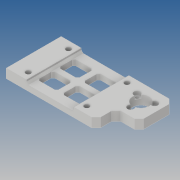
# Autodesk Inventor part: attache_moteur
Saved by Autodesk Inventor 2019 (Build 230136000, 136)
## iProperties
Created: 2020-07-07
Part Number: attache_moteur
Material: Générique
Document SubType Name: Modeling
Designer: Theo
Density: 1 g/cm^3
Appearance: Par défaut
Author: Theo
Autodesk Inventor part; units mm, degrees
ref_plane "YZ Plane" through (0, 0, 0) normal (1, 0, 0) x (0, 1, 0)
ref_plane "XZ Plane" through (0, 0, 0) normal (0, 1, 0) x (-1, 0, 0)
ref_plane "XY Plane" through (0, 0, 0) normal (0, 0, 1) x (1, 0, 0)
sketch "Esquisse1" plane through (0, 0, 0) normal (0, 1, 0) x (-1, 0, 0)
  line L0 (0, 0) -> (123, 0)
  line L1 (123, 0) -> (123, 60)
  line L2 (123, 60) -> (0, 60)
  line L3 (0, 60) -> (0, 0)
  dimension "d1" = 123
  dimension "d2" = 60
  constraints: 8 end point, 2 parallel, 1 horizontal, 1 perpendicular
  measures "d1" distance of L0.start L0.end
  measures "d2" distance of L2.end L0.start
extrude "Extrusion1" add sketch "Esquisse1" along normal blind 10
sketch "Esquisse2" plane through (0, 10, 0) normal (0, 1, 0) x (1, 0, 0)
  circle A0 centre (-18, -18) radius 9
  line L0 (0, 0) -> (-123, 0) projected
  line L1 (-123, 0) -> (-123, -60) projected
  line L2 (-123, -60) -> (0, -60) projected
  line L3 (0, -60) -> (0, 0) projected
  line L4 (-29, -9) -> (-7, -9) construction
  line L5 (-7, -9) -> (-7, -56) construction
  line L6 (-7, -56) -> (-29, -56) construction
  line L7 (-29, -56) -> (-29, -9) construction
  dimension "d5" = 18
  dimension "d7" = 18
  dimension "d9" = 18
  dimension "d27" = 22
  dimension "d28" = 11
  dimension "d29" = 9
  dimension "d30" = 47
  dimension "d31" = 7
  dimension "d44" = 9
  constraints: 8 end point, 2 parallel, 1 centre point, 1 horizontal, 1 perpendicular
  measures "d5" diameter of A0
  measures "d7" distance from line of L3 A0.centre
  measures "d9" distance from line of A0.centre L0
  measures "d27" distance of L4.start L4.end
  measures "d28" horizontal distance of L4.end A0.centre
  measures "d29" distance from line of L4 A0.centre
  measures "d30" distance of L6.end L4.start
  measures "d31" distance between parallel lines of L3 L5
  measures "d44" distance between parallel lines of L0 L4
extrude "Extrusion2" cut sketch "Esquisse2" against normal up to surface (10 mm away) contours A0
sketch "Esquisse4" plane through (0, 10, 0) normal (0, 1, 0) x (1, 0, 0)
  circle A0 centre (-18, -18) radius 9 projected
  line L0 (0, 0) -> (-123, 0) projected
  line L1 (-123, 0) -> (-123, -60) projected
  line L2 (-123, -60) -> (0, -60) projected
  line L3 (0, -60) -> (0, 0) projected
  point P0 (-18, -29)
  dimension "d16" = 11
  constraints: 1 vertical alignment
  measures "d16" distance of point (-18, -29) A0.centre
hole "Perçage1" at (-18, 10, 29) direction (0, -1, 0) diameter 3.4 end through all counterbore diameter 7 counterbore depth 4 clearance for "Vis d'assemblage à tête hexagonale ISO 24017" size "M3" standard "ISO"
pattern_circular "Réseau circulaire1" count 3 over 360 about axis through (-18, 10, 18) along (0, -1, 0) of "Perçage1"
sketch "Esquisse5" plane through (0, 10, 0) normal (0, 1, 0) x (1, 0, 0)
  arc A0 (-9.2451, -15.9139) -> (-11.816, -11.4611) centre (-8.4737, -12.5) ccw projected
  arc A1 (-15.4291, -26.625) -> (-9.2451, -15.9139) centre (-18, -18) ccw projected
  arc A2 (-20.5709, -26.625) -> (-15.4291, -26.625) centre (-18, -29) ccw projected
  arc A3 (-26.7549, -15.9139) -> (-20.5709, -26.625) centre (-18, -18) ccw projected
  arc A4 (-24.184, -11.4611) -> (-26.7549, -15.9139) centre (-27.5263, -12.5) ccw projected
  arc A5 (-11.816, -11.4611) -> (-24.184, -11.4611) centre (-18, -18) ccw projected
  line L0 (0, 0) -> (-123, 0) projected
  line L1 (-123, 0) -> (-123, -60) projected
  line L2 (-123, -60) -> (0, -60) projected
  line L3 (0, -60) -> (0, 0) projected
  line L4 (-29, -18.7209) -> (-29, -39.8718) construction
  point P0 (-43, -8)
  point P1 (-43, -52)
  point P2 (-107, -8)
  point P3 (-107, -52)
  dimension "d32" = 11
  dimension "d33" = 14
  dimension "d34" = 8
  dimension "d35" = 8
  dimension "d36" = 16
  constraints: 2 end point, 2 horizontal alignment, 2 vertical alignment, 1 vertical
  measures "d32" distance from line of L4 A1.centre
  measures "d33" distance from line of point (-43, -8) L4
  measures "d34" distance from line of L0 point (-43, -8)
  measures "d35" distance from line of L2 point (-43, -52)
  measures "d36" distance from line of L1 point (-107, -8)
hole "Perçage2" at (-43, 10, 8) at (-43, 10, 52) at (-107, 10, 8) at (-107, 10, 52) direction (0, -1, 0) diameter 5.5 end through all clearance for "Vis d'assemblage à tête hexagonale ISO 24017" size "M5" standard "ISO"
sketch "Esquisse6" plane through (0, 10, 0) normal (0, 1, 0) x (1, 0, 0)
  circle A0 centre (-107, -8) radius 2.75 projected
  circle A1 centre (-43, -8) radius 2.75 projected
  circle A2 centre (-43, -52) radius 2.75 projected
  circle A3 centre (-107, -52) radius 2.75 projected
  arc A4 (-9.2451, -15.9139) -> (-11.816, -11.4611) centre (-8.4737, -12.5) ccw projected
  arc A5 (-15.4291, -26.625) -> (-9.2451, -15.9139) centre (-18, -18) ccw projected
  arc A6 (-20.5709, -26.625) -> (-15.4291, -26.625) centre (-18, -29) ccw projected
  arc A7 (-26.7549, -15.9139) -> (-20.5709, -26.625) centre (-18, -18) ccw projected
  arc A8 (-24.184, -11.4611) -> (-26.7549, -15.9139) centre (-27.5263, -12.5) ccw projected
  arc A9 (-11.816, -11.4611) -> (-24.184, -11.4611) centre (-18, -18) ccw projected
  line L0 (0, 0) -> (-123, 0) projected
  line L1 (-123, 0) -> (-123, -60) projected
  line L2 (-123, -60) -> (0, -60) projected
  line L3 (0, -60) -> (0, 0) projected
  line L4 (-99, -10) -> (-78, -10)
  line L5 (-78, -10) -> (-78, -27)
  line L6 (-78, -27) -> (-99, -27)
  line L7 (-99, -27) -> (-99, -10)
  line L8 (-72, -10) -> (-51, -10)
  line L9 (-51, -10) -> (-51, -27)
  line L10 (-51, -27) -> (-72, -27)
  line L11 (-72, -27) -> (-72, -10)
  line L12 (-72, -33) -> (-51, -33)
  line L13 (-51, -33) -> (-51, -50)
  line L14 (-51, -50) -> (-72, -50)
  line L15 (-72, -50) -> (-72, -33)
  line L16 (-99, -33) -> (-78, -33)
  line L17 (-78, -33) -> (-78, -50)
  line L18 (-78, -50) -> (-99, -50)
  line L19 (-99, -50) -> (-99, -33)
  dimension "d47" = 10
  dimension "d48" = 10
  dimension "d49" = 8
  dimension "d50" = 6
  dimension "d51" = 6
  dimension "d52" = 8
  constraints: 32 end point, 8 parallel, 6 point on line, 4 horizontal, 4 perpendicular, 2 collinear, 2 horizontal alignment, 2 vertical alignment
  measures "d47" distance between parallel lines of L0 L4
  measures "d48" distance between parallel lines of L2 L18
  measures "d49" distance from line of L7 A0.centre
  measures "d50" distance between parallel lines of L6 L16
  measures "d51" distance between parallel lines of L11 L5
  measures "d52" distance from line of L9 A1.centre
extrude "Extrusion4" cut sketch "Esquisse6" against normal up to surface (10 mm away) contours L4 L5 L6 L7 | L8 L9 L10 L11 | L12 L13 L14 L15 | L16 L17 L18 L19
chamfer "Chanfrein1" distance 2 angle 45 16 edges at (-78, 5, 27) (-78, 5, 50) (-51, 5, 50) (-51, 5, 27) (-72, 5, 33) (-72, 5, 10) (-99, 5, 10) (-99, 5, 33) (-78, 5, 33) (-78, 5, 10) (-51, 5, 10) (-51, 5, 33) (-99, 5, 50) (-72, 5, 50) (-99, 5, 27) (-72, 5, 27)
chamfer "Chanfrein3" distance 5 angle 45 1 edges at (0, 5, 0)
sketch "Esquisse7" plane through (0, 10, 0) normal (0, 1, 0) x (1, 0, 0)
  line L0 (-5, 0) -> (-123, 0) projected
  line L1 (-101, 0) -> (-49, 0)
  line L2 (-49, 0) -> (-49, -60)
  line L3 (-49, -60) -> (-101, -60)
  line L4 (-101, -60) -> (-101, 0)
  line L5 (-51, -35) -> (-51, -48) projected
  line L6 (-53, -50) -> (-51, -48) projected
  line L7 (-53, -50) -> (-70, -50) projected
  line L8 (-72, -48) -> (-70, -50) projected
  line L9 (-72, -48) -> (-72, -35) projected
  line L10 (-70, -33) -> (-72, -35) projected
  line L11 (-70, -33) -> (-53, -33) projected
  line L12 (-51, -35) -> (-53, -33) projected
  line L13 (-80, -50) -> (-97, -50) projected
  line L14 (-99, -48) -> (-97, -50) projected
  line L15 (-99, -48) -> (-99, -35) projected
  line L16 (-97, -33) -> (-99, -35) projected
  line L17 (-97, -33) -> (-80, -33) projected
  line L18 (-78, -35) -> (-80, -33) projected
  line L19 (-78, -35) -> (-78, -48) projected
  line L20 (-80, -50) -> (-78, -48) projected
  line L21 (-51, -12) -> (-51, -25) projected
  line L22 (-53, -27) -> (-51, -25) projected
  line L23 (-53, -27) -> (-70, -27) projected
  line L24 (-72, -25) -> (-70, -27) projected
  line L25 (-72, -25) -> (-72, -12) projected
  line L26 (-70, -10) -> (-72, -12) projected
  line L27 (-70, -10) -> (-53, -10) projected
  line L28 (-51, -12) -> (-53, -10) projected
  line L29 (-80, -27) -> (-97, -27) projected
  line L30 (-99, -25) -> (-97, -27) projected
  line L31 (-99, -25) -> (-99, -12) projected
  line L32 (-97, -10) -> (-99, -12) projected
  line L33 (-97, -10) -> (-80, -10) projected
  line L34 (-78, -12) -> (-80, -10) projected
  line L35 (-78, -12) -> (-78, -25) projected
  line L36 (-80, -27) -> (-78, -25) projected
  circle A0 centre (-107, -8) radius 2.75 projected
  circle A1 centre (-43, -8) radius 2.75 projected
  circle A2 centre (-43, -52) radius 2.75 projected
  circle A3 centre (-107, -52) radius 2.75 projected
  arc A4 (-9.2451, -15.9139) -> (-11.816, -11.4611) centre (-8.4737, -12.5) ccw projected
  arc A5 (-15.4291, -26.625) -> (-9.2451, -15.9139) centre (-18, -18) ccw projected
  arc A6 (-20.5709, -26.625) -> (-15.4291, -26.625) centre (-18, -29) ccw projected
  arc A7 (-26.7549, -15.9139) -> (-20.5709, -26.625) centre (-18, -18) ccw projected
  arc A8 (-24.184, -11.4611) -> (-26.7549, -15.9139) centre (-27.5263, -12.5) ccw projected
  arc A9 (-11.816, -11.4611) -> (-24.184, -11.4611) centre (-18, -18) ccw projected
  line L37 (0, -60) -> (0, -5) projected
  line L38 (-5, 0) -> (0, -5) projected
  line L39 (-5, 0) -> (-123, 0) projected
  line L40 (-123, 0) -> (-123, -60) projected
  line L41 (-123, -60) -> (0, -60) projected
  line L42 (-123, -60) -> (-25, -60) projected
  point P0 (0, 0)
  dimension "d67" = 6
  dimension "d68" = 6
  constraints: 8 end point, 2 parallel, 2 point on line, 1 horizontal, 1 perpendicular
  measures "d67" distance from line of L2 A1.centre
  measures "d68" distance from line of A0.centre L4
extrude "Extrusion5" cut sketch "Esquisse7" against normal blind 4 contours L2 L3 L4 L0
chamfer "Chanfrein5" distance 2 angle 45 2 edges at (-101, 6, 30) (-49, 6, 30)
sketch "Esquisse8" plane through (0, 10, 0) normal (0, 1, 0) x (1, 0, 0)
  line L0 (-123, -60) -> (0, -60) projected
  line L1 (0, -60) -> (-25, -60)
  line L2 (-25, -60) -> (-25, -38)
  line L3 (-25, -38) -> (0, -38)
  line L4 (0, -38) -> (0, -60)
  point P0 (0, 0)
  dimension "d74" = 25
  dimension "d75" = 22
  constraints: 8 end point, 2 parallel, 1 horizontal, 1 perpendicular
  measures "d74" distance of L2.end L3.end
  measures "d75" distance of L3.end L0.end
extrude "Extrusion6" cut sketch "Esquisse8" against normal up to surface (10 mm away)
chamfer "Chanfrein6" distance 5 angle 45 3 edges at (-25, 5, 38) (-25, 5, 60) (0, 5, 38)
equation "\"d28\" = 0.5 * d27"
equation "\"d35\" = d34"
equation "\"d51\" = d50"
